Autodesk Inventor part; units mm, degrees
(part 3 of 3)
sketch "Sketch40" plane through (0, 40.64, 196.85) normal (1, 0, 0) x (0, 0, -1)
  circle A0 centre (98.425, -10.16) radius 2.54
  circle A1 centre (84.455, -18.415) radius 1.905
  circle A2 centre (112.395, -18.415) radius 1.905
  line L0 (91.821, -21.59) -> (91.821, -15.24)
  line L1 (91.821, -15.24) -> (105.029, -15.24)
  line L2 (105.029, -15.24) -> (105.029, -21.59)
  line L3 (105.029, -21.59) -> (91.821, -21.59)
  line L4 (196.85, -30.48) -> (0, -30.48)
  line L5 (196.85, -30.48) -> (196.85, 0)
  line L6 (0, 0) -> (196.85, 0)
  line L7 (0, -30.48) -> (0, 0)
  line L8 (4.7625, -27.94) -> (7.9375, -22.440739)
  line L9 (7.9375, -22.440739) -> (11.1125, -27.94)
  line L10 (11.1125, -27.94) -> (4.7625, -27.94)
  line L11 (14.2875, -27.94) -> (17.4625, -22.440739)
  line L12 (17.4625, -22.440739) -> (20.6375, -27.94)
  line L13 (20.6375, -27.94) -> (14.2875, -27.94)
  line L14 (23.8125, -27.94) -> (26.9875, -22.440739)
  line L15 (26.9875, -22.440739) -> (30.1625, -27.94)
  line L16 (30.1625, -27.94) -> (23.8125, -27.94)
  line L17 (33.3375, -27.94) -> (36.5125, -22.440739)
  line L18 (36.5125, -22.440739) -> (39.6875, -27.94)
  line L19 (39.6875, -27.94) -> (33.3375, -27.94)
  line L20 (42.8625, -27.94) -> (46.0375, -22.440739)
  line L21 (46.0375, -22.440739) -> (49.2125, -27.94)
  line L22 (49.2125, -27.94) -> (42.8625, -27.94)
  line L23 (52.3875, -27.94) -> (55.5625, -22.440739)
  line L24 (55.5625, -22.440739) -> (58.7375, -27.94)
  line L25 (58.7375, -27.94) -> (52.3875, -27.94)
  line L26 (61.9125, -27.94) -> (65.0875, -22.440739)
  line L27 (65.0875, -22.440739) -> (68.2625, -27.94)
  line L28 (68.2625, -27.94) -> (61.9125, -27.94)
  line L29 (71.4375, -27.94) -> (74.6125, -22.440739)
  line L30 (74.6125, -22.440739) -> (77.7875, -27.94)
  line L31 (77.7875, -27.94) -> (71.4375, -27.94)
  line L32 (80.9625, -27.94) -> (84.1375, -22.440739)
  line L33 (84.1375, -22.440739) -> (87.3125, -27.94)
  line L34 (87.3125, -27.94) -> (80.9625, -27.94)
  line L35 (90.4875, -27.94) -> (93.6625, -22.440739)
  line L36 (93.6625, -22.440739) -> (96.8375, -27.94)
  line L37 (96.8375, -27.94) -> (90.4875, -27.94)
  line L38 (100.0125, -27.94) -> (103.1875, -22.440739)
  line L39 (103.1875, -22.440739) -> (106.3625, -27.94)
  line L40 (106.3625, -27.94) -> (100.0125, -27.94)
  line L41 (109.5375, -27.94) -> (112.7125, -22.440739)
  line L42 (112.7125, -22.440739) -> (115.8875, -27.94)
  line L43 (115.8875, -27.94) -> (109.5375, -27.94)
  line L44 (119.0625, -27.94) -> (122.2375, -22.440739)
  line L45 (122.2375, -22.440739) -> (125.4125, -27.94)
  line L46 (125.4125, -27.94) -> (119.0625, -27.94)
  line L47 (128.5875, -27.94) -> (131.7625, -22.440739)
  line L48 (131.7625, -22.440739) -> (134.9375, -27.94)
  line L49 (134.9375, -27.94) -> (128.5875, -27.94)
  line L50 (138.1125, -27.94) -> (141.2875, -22.440739)
  line L51 (141.2875, -22.440739) -> (144.4625, -27.94)
  line L52 (144.4625, -27.94) -> (138.1125, -27.94)
  line L53 (147.6375, -27.94) -> (150.8125, -22.440739)
  line L54 (150.8125, -22.440739) -> (153.9875, -27.94)
  line L55 (153.9875, -27.94) -> (147.6375, -27.94)
  line L56 (157.1625, -27.94) -> (160.3375, -22.440739)
  line L57 (160.3375, -22.440739) -> (163.5125, -27.94)
  line L58 (163.5125, -27.94) -> (157.1625, -27.94)
  line L59 (166.6875, -27.94) -> (169.8625, -22.440739)
  line L60 (169.8625, -22.440739) -> (173.0375, -27.94)
  line L61 (173.0375, -27.94) -> (166.6875, -27.94)
  line L62 (176.2125, -27.94) -> (179.3875, -22.440739)
  line L63 (179.3875, -22.440739) -> (182.5625, -27.94)
  line L64 (182.5625, -27.94) -> (176.2125, -27.94)
  line L65 (185.7375, -27.94) -> (188.9125, -22.440739)
  line L66 (188.9125, -22.440739) -> (192.0875, -27.94)
  line L67 (192.0875, -27.94) -> (185.7375, -27.94)
  line L68 (4.7625, -18.415) -> (7.9375, -12.915739)
  line L69 (7.9375, -12.915739) -> (11.1125, -18.415)
  line L70 (11.1125, -18.415) -> (4.7625, -18.415)
  line L71 (14.2875, -18.415) -> (17.4625, -12.915739)
  line L72 (17.4625, -12.915739) -> (20.6375, -18.415)
  line L73 (20.6375, -18.415) -> (14.2875, -18.415)
  line L74 (23.8125, -18.415) -> (26.9875, -12.915739)
  line L75 (26.9875, -12.915739) -> (30.1625, -18.415)
  line L76 (30.1625, -18.415) -> (23.8125, -18.415)
  line L77 (33.3375, -18.415) -> (36.5125, -12.915739)
  line L78 (36.5125, -12.915739) -> (39.6875, -18.415)
  line L79 (39.6875, -18.415) -> (33.3375, -18.415)
  line L80 (42.8625, -18.415) -> (46.0375, -12.915739)
  line L81 (46.0375, -12.915739) -> (49.2125, -18.415)
  line L82 (49.2125, -18.415) -> (42.8625, -18.415)
  line L83 (52.3875, -18.415) -> (55.5625, -12.915739)
  line L84 (55.5625, -12.915739) -> (58.7375, -18.415)
  line L85 (58.7375, -18.415) -> (52.3875, -18.415)
  line L86 (61.9125, -18.415) -> (65.0875, -12.915739)
  line L87 (65.0875, -12.915739) -> (68.2625, -18.415)
  line L88 (68.2625, -18.415) -> (61.9125, -18.415)
  line L89 (71.4375, -18.415) -> (74.6125, -12.915739)
  line L90 (74.6125, -12.915739) -> (77.7875, -18.415)
  line L91 (77.7875, -18.415) -> (71.4375, -18.415)
  line L92 (80.9625, -18.415) -> (84.1375, -12.915739)
  line L93 (84.1375, -12.915739) -> (87.3125, -18.415)
  line L94 (87.3125, -18.415) -> (80.9625, -18.415)
  line L95 (90.4875, -18.415) -> (93.6625, -12.915739)
  line L96 (93.6625, -12.915739) -> (96.8375, -18.415)
  line L97 (96.8375, -18.415) -> (90.4875, -18.415)
  line L98 (100.0125, -18.415) -> (103.1875, -12.915739)
  line L99 (103.1875, -12.915739) -> (106.3625, -18.415)
  line L100 (106.3625, -18.415) -> (100.0125, -18.415)
  line L101 (109.5375, -18.415) -> (112.7125, -12.915739)
  line L102 (112.7125, -12.915739) -> (115.8875, -18.415)
  line L103 (115.8875, -18.415) -> (109.5375, -18.415)
  line L104 (119.0625, -18.415) -> (122.2375, -12.915739)
  line L105 (122.2375, -12.915739) -> (125.4125, -18.415)
  line L106 (125.4125, -18.415) -> (119.0625, -18.415)
  line L107 (128.5875, -18.415) -> (131.7625, -12.915739)
  line L108 (131.7625, -12.915739) -> (134.9375, -18.415)
  line L109 (134.9375, -18.415) -> (128.5875, -18.415)
  line L110 (138.1125, -18.415) -> (141.2875, -12.915739)
  line L111 (141.2875, -12.915739) -> (144.4625, -18.415)
  line L112 (144.4625, -18.415) -> (138.1125, -18.415)
  line L113 (147.6375, -18.415) -> (150.8125, -12.915739)
  line L114 (150.8125, -12.915739) -> (153.9875, -18.415)
  line L115 (153.9875, -18.415) -> (147.6375, -18.415)
  line L116 (157.1625, -18.415) -> (160.3375, -12.915739)
  line L117 (160.3375, -12.915739) -> (163.5125, -18.415)
  line L118 (163.5125, -18.415) -> (157.1625, -18.415)
  line L119 (166.6875, -18.415) -> (169.8625, -12.915739)
  line L120 (169.8625, -12.915739) -> (173.0375, -18.415)
  line L121 (173.0375, -18.415) -> (166.6875, -18.415)
  line L122 (176.2125, -18.415) -> (179.3875, -12.915739)
  line L123 (179.3875, -12.915739) -> (182.5625, -18.415)
  line L124 (182.5625, -18.415) -> (176.2125, -18.415)
  line L125 (185.7375, -18.415) -> (188.9125, -12.915739)
  line L126 (188.9125, -12.915739) -> (192.0875, -18.415)
  line L127 (192.0875, -18.415) -> (185.7375, -18.415)
  line L128 (4.7625, -8.89) -> (7.9375, -3.390739)
  line L129 (7.9375, -3.390739) -> (11.1125, -8.89)
  line L130 (11.1125, -8.89) -> (4.7625, -8.89)
  line L131 (14.2875, -8.89) -> (17.4625, -3.390739)
  line L132 (17.4625, -3.390739) -> (20.6375, -8.89)
  line L133 (20.6375, -8.89) -> (14.2875, -8.89)
  line L134 (23.8125, -8.89) -> (26.9875, -3.390739)
  line L135 (26.9875, -3.390739) -> (30.1625, -8.89)
  line L136 (30.1625, -8.89) -> (23.8125, -8.89)
  line L137 (33.3375, -8.89) -> (36.5125, -3.390739)
  line L138 (36.5125, -3.390739) -> (39.6875, -8.89)
  line L139 (39.6875, -8.89) -> (33.3375, -8.89)
  line L140 (42.8625, -8.89) -> (46.0375, -3.390739)
  line L141 (46.0375, -3.390739) -> (49.2125, -8.89)
  line L142 (49.2125, -8.89) -> (42.8625, -8.89)
  line L143 (52.3875, -8.89) -> (55.5625, -3.390739)
  line L144 (55.5625, -3.390739) -> (58.7375, -8.89)
  line L145 (58.7375, -8.89) -> (52.3875, -8.89)
  line L146 (61.9125, -8.89) -> (65.0875, -3.390739)
  line L147 (65.0875, -3.390739) -> (68.2625, -8.89)
  line L148 (68.2625, -8.89) -> (61.9125, -8.89)
  line L149 (71.4375, -8.89) -> (74.6125, -3.390739)
  line L150 (74.6125, -3.390739) -> (77.7875, -8.89)
  line L151 (77.7875, -8.89) -> (71.4375, -8.89)
  line L152 (80.9625, -8.89) -> (84.1375, -3.390739)
  line L153 (84.1375, -3.390739) -> (87.3125, -8.89)
  line L154 (87.3125, -8.89) -> (80.9625, -8.89)
  line L155 (90.4875, -8.89) -> (93.6625, -3.390739)
  line L156 (93.6625, -3.390739) -> (96.8375, -8.89)
  line L157 (96.8375, -8.89) -> (90.4875, -8.89)
  line L158 (100.0125, -8.89) -> (103.1875, -3.390739)
  line L159 (103.1875, -3.390739) -> (106.3625, -8.89)
  line L160 (106.3625, -8.89) -> (100.0125, -8.89)
  line L161 (109.5375, -8.89) -> (112.7125, -3.390739)
  line L162 (112.7125, -3.390739) -> (115.8875, -8.89)
  line L163 (115.8875, -8.89) -> (109.5375, -8.89)
  line L164 (119.0625, -8.89) -> (122.2375, -3.390739)
  line L165 (122.2375, -3.390739) -> (125.4125, -8.89)
  line L166 (125.4125, -8.89) -> (119.0625, -8.89)
  line L167 (128.5875, -8.89) -> (131.7625, -3.390739)
  line L168 (131.7625, -3.390739) -> (134.9375, -8.89)
  line L169 (134.9375, -8.89) -> (128.5875, -8.89)
  line L170 (138.1125, -8.89) -> (141.2875, -3.390739)
  line L171 (141.2875, -3.390739) -> (144.4625, -8.89)
  line L172 (144.4625, -8.89) -> (138.1125, -8.89)
  line L173 (147.6375, -8.89) -> (150.8125, -3.390739)
  line L174 (150.8125, -3.390739) -> (153.9875, -8.89)
  line L175 (153.9875, -8.89) -> (147.6375, -8.89)
  line L176 (157.1625, -8.89) -> (160.3375, -3.390739)
  line L177 (160.3375, -3.390739) -> (163.5125, -8.89)
  line L178 (163.5125, -8.89) -> (157.1625, -8.89)
  line L179 (166.6875, -8.89) -> (169.8625, -3.390739)
  line L180 (169.8625, -3.390739) -> (173.0375, -8.89)
  line L181 (173.0375, -8.89) -> (166.6875, -8.89)
  line L182 (176.2125, -8.89) -> (179.3875, -3.390739)
  line L183 (179.3875, -3.390739) -> (182.5625, -8.89)
  line L184 (182.5625, -8.89) -> (176.2125, -8.89)
  line L185 (185.7375, -8.89) -> (188.9125, -3.390739)
  line L186 (188.9125, -3.390739) -> (192.0875, -8.89)
  line L187 (192.0875, -8.89) -> (185.7375, -8.89)
  line L188 (98.425, -10.16) -> (98.425, -30.48) construction
  line L189 (98.425, -10.16) -> (98.425, 0) construction
  point P0 (196.85, -40.64)
  point P1 (95.004413, -15.24)
  point P2 (91.821, -18.415)
  point P3 (91.821, -16.10531)
  point P4 (92.320587, -15.24)
  dimension "d384" = 6.35
  dimension "d385" = 60
  dimension "d388" = 9.525
  dimension "d391" = 9.525
  dimension "d394" = 2.54
  dimension "d395" = 1.5875
  constraints: 364 end point, 2 midpoint, 1 equal length, 1 horizontal, 1 perpendicular, 1 vertical, 354 other
  measures "d384" distance of L9.end L8.start
  measures "d385" angle of L9 L8
  measures "d388" distance of L8.start L11.start
  measures "d391" distance of L8.start L68.start
  measures "d394" distance between parallel lines of L4 L10
  measures "d395" distance from line of L188 L158.start
extrude "Cutouts4" cut sketch "Sketch40" against normal up to surface (3.175 mm away) contours A0 L157 L156 L158 L160 | L160 L158 A0 | A0 L156 L157 | L94 A1 | A1 L94 | L103 A2 | A2 L103 | L0 L97 L96 L1 L98 L100 L2 L3 | L0 L1 L95 | L100 L98 L1 L99 L2 | L99 L1 L2 | L8 L9 L10 | L11 L12 L13 | L14 L15 L16 | L17 L18 L19 | L20 L21 L22 | L23 L24 L25 | L26 L27 L28 | L29 L30 L31 | L32 L33 L34 | L35 L36 L37 | L38 L39 L40 | L41 L42 L43 | L44 L45 L46 | L47 L48 L49 | L50 L51 L52 | L53 L54 L55 | L56 L57 L58 | L59 L60 L61 | L62 L63 L64 | L65 L66 L67 | L68 L69 L70 | L71 L72 L73 | L74 L75 L76 | L77 L78 L79 | L80 L81 L82 | L83 L84 L85 | L86 L87 L88 | L89 L90 L91 | L104 L105 L106 | L107 L108 L109 | L110 L111 L112 | L113 L114 L115 | L116 L117 L118 | L119 L120 L121 | L122 L123 L124 | L125 L126 L127 | L128 L129 L130 | L131 L132 L133 | L134 L135 L136 | L137 L138 L139 | L140 L141 L142 | L143 L144 L145 | L146 L147 L148 | L149 L150 L151 | L152 L153 L154 | L161 L162 L163 | L164 L165 L166 | L167 L168 L169 | L170 L171 L172 | L173 L174 L175 | L176 L177 L178 | L179 L180 L181 | L182 L183 L184 | L185 L186 L187
sketch "Sketch8" plane through (-152.4, 0, 47.625) normal (0, 0, 1) x (1, 0, 0)
  line L0 (-63.5, 10.16) -> (-63.5, 40.64)
  line L1 (-63.5, 31.75) -> (-0.38063, 31.75) construction
  line L2 (-57.15, 50.8) -> (0.781721, 50.8)
  line L3 (-38.1, 63.5) -> (-38.1, 0) construction
  line L4 (-57.15, 0) -> (0, 0)
  line L5 (-50.8, 0) -> (-63.5, 20.32)
  line L6 (-50.8, 0) -> (0, 0)
  line L7 (0, 0) -> (0, 63.5)
  line L8 (-50.8, 63.5) -> (0, 63.5)
  line L9 (-63.5, 43.18) -> (-50.8, 63.5)
  line L10 (-63.5, 20.32) -> (-63.5, 43.18)
  circle A0 centre (-38.1, 31.75) radius 13.127
  arc A1 (-46.85575, 46.073509) -> (-52.423509, 40.50575) centre (-49.639629, 43.289629) ccw
  line L11 (-52.423509, 40.50575) -> (-49.73877, 37.821011)
  line L12 (-46.85575, 46.073509) -> (-44.171011, 43.38877)
  line L13 (-38.1, 31.75) -> (-52.423509, 46.073509) construction
  line L14 (-52.423509, 22.99425) -> (-49.73877, 25.678989)
  line L15 (-38.1, 31.75) -> (-52.423509, 17.426491) construction
  arc A2 (-52.423509, 22.99425) -> (-46.85575, 17.426491) centre (-49.639629, 20.210371) ccw
  line L16 (-46.85575, 17.426491) -> (-44.171011, 20.11123)
  line L17 (-29.34425, 17.426491) -> (-32.028989, 20.11123)
  line L18 (-38.1, 31.75) -> (-23.776491, 17.426491) construction
  arc A3 (-29.34425, 17.426491) -> (-23.776491, 22.99425) centre (-26.560371, 20.210371) ccw
  line L19 (-23.776491, 22.99425) -> (-26.46123, 25.678989)
  line L20 (-23.776491, 40.50575) -> (-26.46123, 37.821011)
  line L21 (-38.1, 31.75) -> (-23.776491, 46.073509) construction
  arc A4 (-23.776491, 40.50575) -> (-29.34425, 46.073509) centre (-26.560371, 43.289629) ccw
  line L22 (-29.34425, 46.073509) -> (-32.028989, 43.38877)
  point P0 (152.4, 0)
  point P1 (0.781721, 50.8)
  point P2 (-49.73877, 25.678989)
  point P3 (-44.171011, 20.11123)
  point P4 (-32.028989, 20.11123)
  point P5 (-26.46123, 25.678989)
  point P6 (-26.46123, 37.821011)
  dimension "d60" = 25.4
  dimension "d61" = 26.254
  dimension "d62" = 7.874
  dimension "d63" = 45
  dimension "d64" = 16.3195
  dimension "d67" = 360
  constraints: 28 end point, 11 point on circle, 5 centre point, 2 coincident, 2 parallel, 2 point on line, 2 tangent, 1 horizontal, 1 midpoint, 1 vertical, 45 other
  measures "d60" distance between parallel lines of L3 L0
  measures "d61" diameter of A0
  measures "d62" diameter of A1
  measures "d63" angle of L1 L13
  measures "d64" distance of L13.start A1.centre
equation "\"d19\" = d18"
equation "\"d21\" = 0.5 * d15"
equation "\"d24\" = Wall_Thickness"
equation "\"d25\" = Wall_Thickness"
equation "\"d26\" = Wall_Thickness"
equation "\"d29\" = 0.5 * Wall_Thickness"
equation "\"d30\" = 0.5 * Wall_Thickness"
equation "\"d31\" = 0.5 * Wall_Thickness"
equation "\"d46\" = 0.5 * Wall_Height"
equation "\"d18\" = Wall_Thickness"
equation "\"Wall_Thickness\" = 3.175"
equation "\"Wall_Height\" = 50.8"
equation "\"Wheel_Hole_Diameter\" = 79.375"
equation "\"Driven_Wheel_Width\" = 23.495"
equation "\"Brushless_Diameter\" = 26"
body "Solid1"
